Aufsatzscheibe_v1 (Autodesk Fusion 360 design; units mm, degrees)
Autodesk Fusion 360 part; units mm, degrees
sketch "Skizze1" plane through (0, 0, 0) normal (0, 1, 0) x (1, 0, 0)
  circle A0 centre (0, 0) radius 45
  dimension "d1" = 90
  constraint coincident A0.centre origin
  measures "d1" diameter of A0
extrude "Extrusion1" add sketch "Skizze1" along normal blind 7
cylinder "Grundkörper Zylinder1" cut diameter 5.5 height -10 placed x (1, 0, 0) y (0, 0, -1) z (0, 1, 0) at (0, 7, 0)
cylinder "Grundkörper Zylinder2" cut diameter 10 height -5 placed x (1, 0, 0) y (0, 0, -1) z (0, 1, 0) at (0, 7, 0)
fillet "Abrundung1" radius 1 2 edges at (-41.9547, 0, 16.2727) (-41.9547, 7, 16.2727)
fillet "Abrundung2" radius 0.3 2 edges at (0.9944, 0, 2.5639) (0.9944, 2, 2.5639)
fillet "Abrundung3" radius 0.7 1 edges at (-1.8081, 7, 4.6616)
